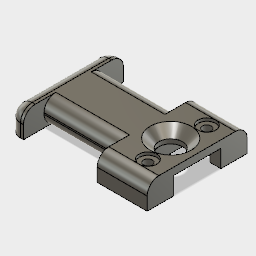
tof-case v2 (Autodesk Fusion 360 design; units mm, degrees)
Autodesk Fusion 360 part; units mm, degrees
sketch "Sketch1" plane through (0, 0, 0) normal (0, 1, 0) x (1, 0, 0)
  line L0 (6, 8) -> (6, -8)
  line L1 (-6, -8) -> (-6, 8)
  circle A0 centre (0.2743, -9.9995) radius 1.5
  circle A1 centre (0.2743, 10) radius 1.5
  circle A2 centre (-2, 0) radius 4
  line L2 (7, 17) -> (-40, 17)
  line L3 (-40, 17) -> (-40, -17)
  line L4 (-40, -17) -> (7, -17)
  line L5 (7, -17) -> (7, 17)
  line L6 (-35, -17) -> (-10, -17)
  line L7 (-10, -17) -> (-10, -10)
  line L8 (-10, -10) -> (-35, -10)
  line L9 (-35, -10) -> (-35, -17)
  line L10 (-10, 17) -> (-35, 17)
  line L11 (-35, 17) -> (-35, 10)
  line L12 (-35, 10) -> (-10, 10)
  line L13 (-10, 10) -> (-10, 17)
  line L14 (6, -8) -> (3.2743, -8)
  arc A3 (-2.7257, -10) -> (3.2743, -10) centre (0.2743, -9.9995) ccw
  arc A4 (3.2743, 10) -> (-2.7257, 10) centre (0.2743, 10) ccw
  line L15 (3.2743, 8) -> (6, 8)
  line L16 (-2.7257, -8) -> (-6, -8)
  line L17 (-1.9623, -8) -> (-2.7257, -8)
  line L18 (-6, 8) -> (-2.7257, 8)
  line L19 (-2.7257, 8) -> (-2.7257, 10)
  line L20 (3.2743, 10) -> (3.2743, 8)
  line L21 (-2.7257, -10) -> (-2.7257, -8)
  line L22 (3.2743, -10) -> (3.2743, -8)
  line L23 (7, -8) -> (4.5, -8)
  line L24 (4.5, -8) -> (4.5, 8)
  line L25 (4.5, 8) -> (7, 8)
  line L26 (7, 8) -> (7, -8)
  dimension "d2" = 3
  dimension "d3" = 3
  measures "d2" diameter of A0
  measures "d3" diameter of A1
extrude "Extrude1" add sketch "Sketch1" along normal blind 8.5 contours L0 L5 L23 L25 L26 | L1 L2 L3 L4 L5 L7 L8 L9 L11 L12 L13 L14 A3 A4 L15 L16 L18 L19 L20 L21 L22 L23 L25
fillet "Fillet1" radius 4 11 edges at (-22.5, 8.5, -10) (-22.5, 8.5, 10) (-22.5, 0, 10) (-37.5, 8.5, 17) (-40, 8.5, 0) (-37.5, 8.5, -17) (-22.5, 0, -10) (-40, 4.25, -17) (-40, 4.25, 17) (-1.5, 8.5, -17) (-1.5, 8.5, 17)
delete_face "DeleteFace1" 12 faces at (-6, 2.8333, 2.6667) (6, 2.8333, -2.6667) (4.1829, 2.8333, -8) (3.2743, 2.8333, -9.3333) (-2.2856, 2.8333, -11.5643) (3.2743, 5.6667, 8.6667) (2.2592, 2.8333, 12.249) (-4.9086, 2.8333, -8) (-3.8171, 2.8333, 8) (-2.7257, 2.8333, 9.3333) (-2.7257, 2.8333, -8.6667) (5.0914, 2.8333, 8)
extrude "Extrude2" cut sketch "Sketch1" along normal blind 10 contours A0 | A1
extrude "Extrude3" cut sketch "Sketch1" along normal blind 12 contours A2
extrude "Extrude4" cut sketch "Sketch1" along normal blind 4 contours L0 L14 L15 L23 L24 L25 | L1 L14 A3 A4 L15 L16 L18 L19 L20 L21 L22 L24
chamfer "Chamfer1" distance 3 angle 45 1 edges at (-5.7293, 8.5, -1.4465)
hole "Hole2" at (0.2743, 8.5, -10) direction (0, -1, 0) diameter 6 depth 1 tip angle 180
hole "Hole3" at (0.2743, 8.5, 9.9995) direction (0, -1, 0) diameter 6 depth 1 tip angle 180
extrude "Extrude6" cut sketch "Sketch1" along normal blind 6 contours L0 L5 L23 L25 L26
extrude "Extrude7" cut sketch "Sketch1" along normal blind 6 contours L0 L14 L15 L23 L24 L25
boxprimitive "BoxPrimitive1" [rolled back] distance x 6 distance y 16 distance z 1 offset distance x 0 offset distance y 0
